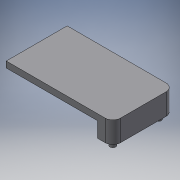
# Autodesk Inventor part: GearCover
Saved by Autodesk Inventor 2019 (Build 230136000, 136)
## iProperties
Created: 2019-08-07
Part Number: GearCover
Material: Generic
Document SubType Name: Modeling
Designer: aorfi
Density: 1 g/cm^3
Appearance: Default
Author: aorfi
Autodesk Inventor part; units mm, degrees
ref_plane "YZ Plane" through (0, 0, 0) normal (1, 0, 0) x (0, 1, 0)
ref_plane "XZ Plane" through (0, 0, 0) normal (0, 1, 0) x (-1, 0, 0)
ref_plane "XY Plane" through (0, 0, 0) normal (0, 0, 1) x (1, 0, 0)
sketch "Sketch1" plane through (0, 0, 0) normal (0, 1, 0) x (-1, 0, 0)
  line L0 (-20, 10) -> (20, 10)
  line L1 (20, 10) -> (20, -10)
  line L2 (20, -10) -> (-20, -10)
  line L3 (-20, -10) -> (-20, 10)
  line L4 (-20, 10) -> (20, -10) construction
  line L5 (20, 10) -> (-20, -10) construction
  point P0 (0, 0)
  dimension "d2" = 40
  dimension "d3" = 20
  constraints: 12 end point, 2 midpoint, 2 parallel, 1 horizontal, 1 perpendicular
  measures "d2" distance of L1.end L2.end
  measures "d3" distance of L2.end L0.start
extrude "Extrusion1" add sketch "Sketch1" along normal mid plane 2
sketch "Sketch5" plane through (0, -1, 0) normal (0, -1, 0) x (1, 0, 0)
  line L0 (20, 10) -> (15, 10)
  line L1 (15, 10) -> (15, -10)
  line L2 (15, -10) -> (20, -10)
  line L3 (20, -10) -> (20, 10)
  line L4 (20, 10) -> (-20, 10) projected
  line L5 (20, -10) -> (20, 10) projected
  line L6 (-20, -10) -> (20, -10) projected
  dimension "d25" = 5
  constraints: 8 end point, 3 collinear, 2 parallel, 1 horizontal, 1 perpendicular
  measures "d25" distance between parallel lines of L3 L1
extrude "Extrusion4" add sketch "Sketch5" along normal blind 5
sketch "Sketch4" plane through (0, -6, 0) normal (0, -1, 0) x (1, 0, 0)
  circle A0 centre (17.5, 7.5) radius 0.95
  circle A1 centre (17.5, -7.5) radius 0.95
  line L0 (20, -10) -> (20, 10) projected
  line L1 (20, 10) -> (15, 10) projected
  line L2 (15, -10) -> (20, -10) projected
  dimension "d26" = 1.9
  dimension "d27" = 1.9
  dimension "d28" = 2.5
  dimension "d29" = 2.5
  dimension "d30" = 2.5
  constraints: 2 centre point, 1 vertical alignment
  measures "d26" diameter of A0
  measures "d27" diameter of A1
  measures "d28" distance from line of L0 A0.centre
  measures "d29" distance from line of L1 A0.centre
  measures "d30" distance from line of L2 A1.centre
extrude "Extrusion3" add sketch "Sketch4" along normal blind 2
sketch "Sketch6" plane through (0, -1, 0) normal (0, -1, 0) x (1, 0, 0)
  circle A0 centre (-18.5, 8) radius 0.95
  circle A1 centre (-18.5, -8) radius 0.95
  line L0 (-20, 10) -> (-20, -10) projected
  line L1 (15, 10) -> (-20, 10) projected
  line L2 (-20, -10) -> (15, -10) projected
  point P0 (0, 0)
  dimension "d31" = 1.9
  dimension "d32" = 1.9
  dimension "d33" = 1.5
  dimension "d34" = 2
  dimension "d35" = 2
  constraints: 2 centre point, 1 vertical alignment
  measures "d31" diameter of A0
  measures "d32" diameter of A1
  measures "d33" distance from line of L0 A0.centre
  measures "d34" distance from line of L1 A0.centre
  measures "d35" distance from line of L2 A1.centre
extrude "Extrusion5" add sketch "Sketch6" along normal blind 2
fillet "Fillet1" radius 2 4 edges at (20, -2.5, 10) (20, -2.5, -10) (-20, 0, 10) (-20, 0, -10)
sketch "Sketch7" plane through (0, 1, 0) normal (0, 1, 0) x (1, 0, 0)
  circle A0 centre (4.677, 0) radius 3.9688 projected
  circle A1 centre (4.677, 0) radius 5.5
  point P0 (0, 0)
  dimension "d38" = 11
  constraints: 1 centre point, 1 coincident
  measures "d38" diameter of A1
extrude "Extrusion6" cut sketch "Sketch7" against normal through all contours A0 | A1
sketch "Sketch8" plane through (0, 1, 0) normal (0, 1, 0) x (1, 0, 0)
  circle A0 centre (-12, 0) radius 2.1525 projected
  point P0 (0, 0)
hole "Hole1" at (-12, 1, 0) direction (0, -1, 0) diameter 4.305 end through all clearance for "Flat Head Machine Screw (82)" size "#6" standard "Ansi Unified Screw Threads"
equation "\"d27\" = d26"
equation "\"d29\" = d28"
equation "\"d30\" = d29"
equation "\"d32\" = d31"
equation "\"d35\" = d34"
body "Solid1"
